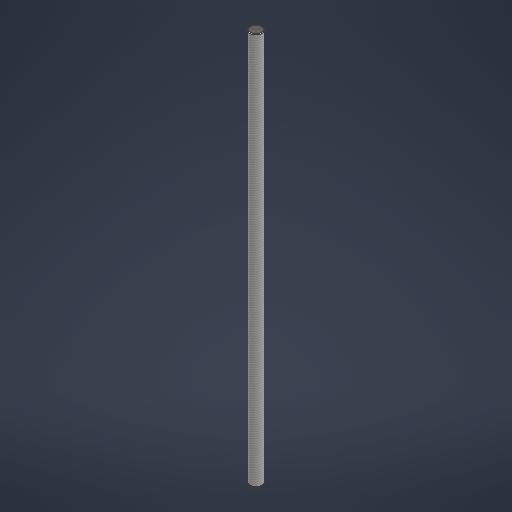
# Autodesk Inventor part: Gewindestange
Saved by Autodesk Inventor 2025.2 (Build 292293000, 293)
## iProperties
Created: 2024-11-15
Part Number: Gewindestange
Material: Generisch
Document SubType Name: Modeling
Designer: Fabian
Density: 1 g/cm^3
Appearance: Stahl - poliert
Author: Fabian
Autodesk Inventor part; units mm, degrees
ref_plane "YZ Plane" through (0, 0, 0) normal (1, 0, 0) x (0, 1, 0)
ref_plane "XZ Plane" through (0, 0, 0) normal (0, 1, 0) x (-1, 0, 0)
ref_plane "XY Plane" through (0, 0, 0) normal (0, 0, 1) x (1, 0, 0)
sketch "Skizze1" plane through (0, 0, 0) normal (0, 1, 0) x (-1, 0, 0)
  circle A0 centre (0, 0) radius 2
  dimension "d0" = 4
  constraints: 1 centre point, 1 coincident
  measures "d0" diameter of A0
extrude "Extrusion1" add sketch "Skizze1" along normal blind 133
thread "Gewinde1" size "M4x0.7" class "6g" standard "ISO Metric profile" full length
chamfer "Fasen1" distance 0.2 angle 45 2 edges at (2, 0, 0) (2, 133, 0)
